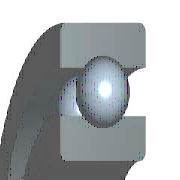
# Autodesk Inventor part: DIN 625 T1 - 619/6 - 6 x 15 x 5
Saved by Autodesk Inventor 2016 (Build 200138000, 138)
## iProperties
IsCustomPart: 0
Created: 2015-02-19
Part Number: DIN 625 T1 - 619/6 - 6 x 15 x 5
Material: Stahl, weich
Description: Rillenkugellager
Document SubType Name: Modeling
Standard: DIN 625 T1
Designer: 4ndreas
Standard Revision: 2011-04
Standards Organization: DIN
Language: de-DE
Size Designation: 619/6 - 6 x 15 x 5
Categories: <MemberInstance><Categories><Category DisplayName="Wellenteile" InternalName="7f7aeb1f-a693-4053-b835-cee3144e0d98" Mnemonic="SHFT"><Category DisplayName="Lager" InternalName="242d30a3-7172-44e6-a363-b0a3d8f1b556" Mnemonic="BRNG"><CategoryParameter DisplayName="Breite" InternalName="25fc5f6e-338b-4801-b5ed-8959743e396e" Mnemonic="wdth"/><CategoryParameter DisplayName="Größenbezeichnung" InternalName="2c4e891a-c8f4-49ed-a5c1-5131476c6feb" Mnemonic="sizedes"/><CategoryParameter DisplayName="Allgemeine Bewertung für dyn. Belastung" InternalName="440972dd-7009-4861-bd45-69ffbb461423" Mnemonic="bdynlrat"/><CategoryParameter DisplayName="Wellendurchmesser" InternalName="91302473-2833-4451-a660-c5d4a8d6a031" Mnemonic="shaftdia"/><CategoryParameter DisplayName="Berührungswinkel" InternalName="aa21a452-7974-4a55-b5cf-1c2972de2aea" Mnemonic="TouchAngle"/><CategoryParameter DisplayName="Außendurchmesser" InternalName="d441686c-04bd-4681-b674-94fbc173ec23" Mnemonic="outdia"/><Category DisplayName="Kugellager" InternalName="9b553946-0899-4a5e-a403-c1d9295e77c1" Mnemonic="BALLBEAR"><CategoryParameter DisplayName="Koeffizient für dynamische Radialbelastung bei Fa/Fr &lt;= e" InternalName="051e59b3-bd55-4dad-8b07-38b5cb912881" Mnemonic="raddynfc1"/><CategoryParameter DisplayName="Allgemeine Bewertung für statische Belastung" InternalName="0f13fbbf-c511-4d43-b4c7-197b47424baf" Mnemonic="bstatlrat"/><CategoryParameter DisplayName="Exponent zur Haltbarkeitsbestimmung" InternalName="3029e2ef-9460-4be8-bdfd-dfe61437473d" Mnemonic="lifeexp"/><CategoryParameter DisplayName="Reibungsfaktor" InternalName="3086b0f2-3d69-46ff-8a75-fe12e395bb47" Mnemonic="fricfct"/><CategoryParameter DisplayName="Min. Wellendurchmesser" InternalName="4a5be9bc-ad86-4bf2-8167-102dad5d3e27" Mnemonic="minshaftdia"/><CategoryParameter DisplayName="Koeffizient für dynamische Axialbelastung bei Fa/Fr &gt; e" InternalName="4b6ff741-5956-4a40-80f5-34eb9259f88c" Mnemonic="axdynfc2"/><CategoryParameter DisplayName="Höchstgeschwindigkeit für Schmierfett" InternalName="5237843b-2c8d-46d3-8227-f3e9dd85a12e" Mnemonic="lubgrsp"/><CategoryParameter DisplayName="Höchstgeschwindigkeit für Öl" InternalName="60628548-8907-44dc-8e09-603d72f5766f" Mnemonic="oilspd"/><CategoryParameter DisplayName="Koeffizient für statische Axialbelastung" InternalName="74dbf5e2-8362-409a-802f-3c2235668d99" Mnemonic="axdynfc0"/><CategoryParameter DisplayName="Masse" InternalName="7b80f85c-da81-4dea-b8db-d7c689da91b2" Mnemonic="mass"/><CategoryParameter DisplayName="Radius" InternalName="83352640-dfae-4cba-bc9f-11ecbfb0001c" Mnemonic="rad"/><CategoryParameter DisplayName="Koeffizient für statische Radialbelastung" InternalName="83ce084d-c51e-4598-a871-e8e1e34b26ee" Mnemonic="raddynfc0"/><CategoryParameter DisplayName="Koeffizient für dynamische Axialbelastung bei Fa/Fr &lt;= e" InternalName="ae45a7db-08df-4411-99a8-2f035015bff9" Mnemonic="axdynfc1"/><CategoryParameter DisplayName="Max. Nabendurchmesser" InternalName="b5cf89e0-ca87-439c-b08c-a25e2999ab06" Mnemonic="maxhubdia"/><CategoryParameter DisplayName="Höchstwert für Faktorbestimmung" InternalName="be0ce6fc-cad4-4218-b484-c34dd2571812" Mnemonic="limvalfac"/><CategoryParameter DisplayName="Koeffizient für dynamische Radialbelastung bei Fa/Fr &gt; e" InternalName="e513bdb7-139f-4b3c-af32-49e0ba1226b9" Mnemonic="raddynfc2"/><CategoryParameter DisplayName="Max. Rundungsradius" InternalName="f6ce6695-cf2c-4ec9-8d20-66671e0e35a4" Mnemonic="maxstprad"/><Category DisplayName="Rillenkugellager" InternalName="6f040212-0f73-4fa8-b5e4-17d6525fdc38" Mnemonic="BBDGBB"/></Category></Category></Category><Category DisplayName="Datentyp" InternalName="23b78d0f-2648-40c6-8793-ca6db495c9e8" Mnemonic="DATATYPE"><CategoryParameter DisplayName="Anzeigename" InternalName="05415f3d-3907-474b-a020-eb9d644f4cf3" Mnemonic="DISPLAYNAME"/><CategoryParameter DisplayName="Norm" InternalName="0c0a119c-1e12-4c84-803f-101930972f5e" Mnemonic="STANDARD"/><CategoryParameter DisplayName="Beschreibung" InternalName="13903e3d-64b1-4950-80da-f627842ea37f" Mnemonic="DESCRIPTION"/><CategoryParameter DisplayName="Bezeichnung" InternalName="2675968c-4ce5-49e0-a4f5-552d29089031" Mnemonic="DESIGNATION"/><CategoryParameter DisplayName="Standardzeile" InternalName="2af9ec52-faaa-4026-b378-f9fa4afca842" Mnemonic="DEFAULTROW"/><CategoryParameter DisplayName="Ordnername" InternalName="3f06958e-8713-4116-9be7-ed6184ecc97b" Mnemonic="FOLDERNAME"/><CategoryParameter DisplayName="Revisionsanleitung" InternalName="45a75005-10b1-4dfc-8d6d-dfe629f0b93c" Mnemonic="REVISIONGUID"/><CategoryParameter DisplayName="Dateiname" InternalName="8b46a4cc-9585-4fed-90c3-899f57e09a73" Mnemonic="FILENAME"/><CategoryParameter DisplayName="Normungsorganisation" InternalName="8f5914e1-4693-403f-8ab5-d37768198c9d" Mnemonic="STDSORG"/><CategoryParameter DisplayName="Gruppenversion" InternalName="914462f6-6e19-4b14-ba84-155b9680b1d0" Mnemonic="FAMILYREVISION"/><CategoryParameter DisplayName="Normrevision" InternalName="91d5a463-65c2-4fde-b823-3b7fea5e8e17" Mnemonic="STANDARDREVISION"/><CategoryParameter DisplayName="Variantenrevision" InternalName="a65d44b9-392f-4f4f-857b-e4b3d54996fe" Mnemonic="MEMBERREVISION"/><CategoryParameter DisplayName="ClipFormat" InternalName="bc51e27b-3422-4e78-93ef-cec197ddf230" Mnemonic="CLIPFORMAT"/><CategoryParameter DisplayName="Hersteller" InternalName="cd6c7a72-a28a-4e50-99a9-2c7f4e13e5ad" Mnemonic="MANUFACTURER"/><CategoryParameter DisplayName="InternerName" InternalName="cf1d0246-76d9-4b4a-8305-fa0409afb5c1" Mnemonic="INTERNALNAME"/><CategoryParameter DisplayName="IstMetrisch" InternalName="e2385c5b-1ea4-4823-96a8-8de651266ec3" Mnemonic="ISMETRIC"/><Category DisplayName="Bauteil" InternalName="c0e0b642-3bcb-4cc8-9e80-f96d35c4afa4" Mnemonic="PART"><CategoryParameter DisplayName="Bauteilnummer" InternalName="016b6077-bfbe-49bd-92c9-d8d59c39c941" Mnemonic="PARTNUMBER"/><CategoryParameter DisplayName="Bestandsnummer" InternalName="4dba7c1c-e26c-444e-836c-b08b433409a8" Mnemonic="STOCKNUMBER"/><CategoryParameter DisplayName="Materialschlüssel" InternalName="5c9a8adb-dd2b-4535-b97f-0a94a95fe41f" Mnemonic="MATERIALKEY"/><CategoryParameter DisplayName="Material" InternalName="818a152a-d3c3-49ca-80ee-df7d91421b8e" Mnemonic="MATERIAL"/></Category></Category><Category DisplayName="ÄltereVersionenzuweisen" InternalName="cd87c42b-3e48-431e-b5c0-1cbeb14dfe77" Mnemonic="LEGACYMAP"><CategoryParameter DisplayName="Eindeutige DA-Varianten-ID" InternalName="0918ad47-427f-4fed-ae26-24c81c58f590" Mnemonic="DACOOKIE"/><CategoryParameter DisplayName="ID zusammenführen" InternalName="0ee8fb18-e2ed-4f39-96f6-1f4b5f50aa71" Mnemonic="MERGE11"/><CategoryParameter DisplayName="Eindeutige CC-Varianten-ID" InternalName="5193edd4-b2b0-4ab4-9d54-de900eee34e0" Mnemonic="CCCOOKIE"/><CategoryParameter DisplayName="ID aufteilen" InternalName="72b5c83c-be7f-45c4-ae51-9160ea6deb26" Mnemonic="SPLIT"/><CategoryParameter DisplayName="VarianteID" InternalName="8e5e0294-fc51-4c8f-b3d7-003dc5ed94f6" Mnemonic="MEMBERID"/><CategoryParameter DisplayName="Katalogname" InternalName="d99d1e27-aa94-4de2-af4c-c348882a6f4f" Mnemonic="CATALOGNAME"/><CategoryParameter DisplayName="Gruppennummer" InternalName="e705e1f4-09cb-413e-91f9-551b4188271e" Mnemonic="FAMILYNUMBER"/></Category></Categories><FamilyTemplate Id="br0026"><FamilyTemplateParameters><FamilyTemplateParameter ObjectType="kUserParameterObject" ValueType="xs:double" Id="1" ObjectReferenceKey="WR"/><FamilyTemplateParameter ObjectType="kUserParameterObject" ValueType="xs:double" Id="2" ObjectReferenceKey="DDB"/><FamilyTemplateParameter ObjectType="kUserParameterObject" ValueType="xs:double" Id="3" ObjectReferenceKey="DDA"/><FamilyTemplateParameter ObjectType="kUserParameterObject" ValueType="xs:double" Id="4" ObjectReferenceKey="KRS"/><FamilyTemplateParameter ObjectType="kUserParameterObject" ValueType="xs:double" Id="5" ObjectReferenceKey="WD"/><FamilyTemplateParameter ObjectType="kUserParameterObject" ValueType="xs:double" Id="6" ObjectReferenceKey="KAD1"/><FamilyTemplateParameter ObjectType="kUserParameterObject" ValueType="xs:double" Id="7" ObjectReferenceKey="KB"/><FamilyTemplateParameter ObjectType="kUserParameterObject" ValueType="xs:double" Id="8" ObjectReferenceKey="BC0"/><FamilyTemplateParameter ObjectType="kUserParameterObject" ValueType="xs:double" Id="9" ObjectReferenceKey="BD"/><FamilyTemplateParameter ObjectType="kUserParameterObject" ValueType="xs:double" Id="10" ObjectReferenceKey="BC"/><FamilyTemplateParameter ObjectType="kUserParameterObject" ValueType="xs:double" Id="11" ObjectReferenceKey="BR"/><FamilyTemplateParameter ObjectType="kUserParameterObject" ValueType="xs:double" Id="12" ObjectReferenceKey="BBA"/><FamilyTemplateParameter ObjectType="kUserParameterObject" ValueType="xs:double" Id="13" ObjectReferenceKey="KID1"/><FamilyTemplateParameter ObjectType="kUserParameterObject" ValueType="xs:double" Id="14" ObjectReferenceKey="BI"/><FamilyTemplateParameter ObjectType="kPropertyObject" ValueType="xs:string" Id="100" ObjectReferenceKey="{32853F0F-3444-11d1-9E93-0060B03C1CA6}" SubObjectId="52"/><FamilyTemplateParameter ObjectType="kPropertyObject" ValueType="xs:string" Id="105" ObjectReferenceKey="{32853F0F-3444-11d1-9E93-0060B03C1CA6}" SubObjectId="5"/><FamilyTemplateParameter ObjectType="kPartComponentDefinitionObject" ValueType="xs:string" Id="110" SubObjectId="Material"/></FamilyTemplateParameters></FamilyTemplate><CategoryParameterMap><ParamToTemplateMap><ParamToTemplate CategoryParameter="//CategoryParameter[@InternalName='05415f3d-3907-474b-a020-eb9d644f4cf3']" ConstantValue="DIN 625 - T1"/><ParamToTemplate CategoryParameter="//CategoryParameter[@InternalName='cf1d0246-76d9-4b4a-8305-fa0409afb5c1']" ConstantValue="5d4a6c16-d65c-4e33-9660-dc348c1d9e25"/><ParamToTemplate CategoryParameter="//CategoryParameter[@InternalName='3f06958e-8713-4116-9be7-ed6184ecc97b']" ConstantValue="DIN 625 - T1"/><ParamToTemplate CategoryParameter="//CategoryParameter[@InternalName='914462f6-6e19-4b14-ba84-155b9680b1d0']" ConstantValue="10"/><ParamToTemplate CategoryParameter="//CategoryParameter[@InternalName='bc51e27b-3422-4e78-93ef-cec197ddf230']" ConstantValue="CF_INVENTOR.STDPARTS"/><ParamToTemplate CategoryParameter="//CategoryParameter[@InternalName='e2385c5b-1ea4-4823-96a8-8de651266ec3']" ConstantValue="true"/><ParamToTemplate CategoryParameter="//CategoryParameter[@InternalName='13903e3d-64b1-4950-80da-f627842ea37f']" ConstantValue="Deep Groove Ball Bearing"/><ParamToTemplate CategoryParameter="//CategoryParameter[@InternalName='8f5914e1-4693-403f-8ab5-d37768198c9d']" ConstantValue="DIN"/><ParamToTemplate CategoryParameter="//CategoryParameter[@InternalName='0c0a119c-1e12-4c84-803f-101930972f5e']" ConstantValue="DIN 625 T1"/><ParamToTemplate CategoryParameter="//CategoryParameter[@InternalName='cd6c7a72-a28a-4e50-99a9-2c7f4e13e5ad']" TemplateParameter="104"/><ParamToTemplate CategoryParameter="//CategoryParameter[@InternalName='91d5a463-65c2-4fde-b823-3b7fea5e8e17']" ConstantValue="2011-04"/><ParamToTemplate CategoryParameter="//CategoryParameter[@InternalName='45a75005-10b1-4dfc-8d6d-dfe629f0b93c']" ConstantValue="d6feace9-0a94-4a7e-876f-687225c7e903"/><ParamToTemplate CategoryParameter="//CategoryParameter[@InternalName='2af9ec52-faaa-4026-b378-f9fa4afca842']" ConstantValue="10"/><ParamToTemplate CategoryParameter="//CategoryParameter[@InternalName='d99d1e27-aa94-4de2-af4c-c348882a6f4f']" ConstantValue="DIN"/><ParamToTemplate CategoryParameter="//CategoryParameter[@InternalName='e705e1f4-09cb-413e-91f9-551b4188271e']" ConstantValue="249"/><ParamToTemplate CategoryParameter="//CategoryParameter[@InternalName='8b46a4cc-9585-4fed-90c3-899f57e09a73']" ConstantValue="DIN 625 T1 - 619/6 - 6 x 15 x 5"/><ParamToTemplate CategoryParameter="//CategoryParameter[@InternalName='a65d44b9-392f-4f4f-857b-e4b3d54996fe']" ConstantValue="51BD74BC-A623-4305-A976-BDE71F3737EF"/><ParamToTemplate CategoryParameter="//CategoryParameter[@InternalName='2c4e891a-c8f4-49ed-a5c1-5131476c6feb']" ConstantValue="619/6"/><ParamToTemplate CategoryParameter="//CategoryParameter[@InternalName='8e5e0294-fc51-4c8f-b3d7-003dc5ed94f6']" ConstantValue="2400"/><ParamToTemplate CategoryParameter="//CategoryParameter[@InternalName='aa21a452-7974-4a55-b5cf-1c2972de2aea']" TemplateParameter="12"/><ParamToTemplate CategoryParameter="//CategoryParameter[@InternalName='440972dd-7009-4861-bd45-69ffbb461423']" TemplateParameter="10"/><ParamToTemplate CategoryParameter="//CategoryParameter[@InternalName='0f13fbbf-c511-4d43-b4c7-197b47424baf']" TemplateParameter="8"/><ParamToTemplate CategoryParameter="//CategoryParameter[@InternalName='d441686c-04bd-4681-b674-94fbc173ec23']" TemplateParameter="9"/><ParamToTemplate CategoryParameter="//CategoryParameter[@InternalName='2675968c-4ce5-49e0-a4f5-552d29089031']" TemplateParameter="100"/><ParamToTemplate CategoryParameter="//CategoryParameter[@InternalName='25fc5f6e-338b-4801-b5ed-8959743e396e']" TemplateParameter="7"/><ParamToTemplate CategoryParameter="//CategoryParameter[@InternalName='83352640-dfae-4cba-bc9f-11ecbfb0001c']" TemplateParameter="4"/><ParamToTemplate CategoryParameter="//CategoryParameter[@InternalName='818a152a-d3c3-49ca-80ee-df7d91421b8e']" TemplateParameter="110"/><ParamToTemplate CategoryParameter="//CategoryParameter[@InternalName='016b6077-bfbe-49bd-92c9-d8d59c39c941']" TemplateParameter="105"/><ParamToTemplate CategoryParameter="//CategoryParameter[@InternalName='91302473-2833-4451-a660-c5d4a8d6a031']" TemplateParameter="5"/></ParamToTemplateMap></CategoryParameterMap></MemberInstance>
Density: 7.85 g/cm^3
Appearance: Halbpoliert
Mass: 1.68915 g
Surface Area: 6.84168 cm^2
Volume: 0.215178 cm^3
Author: 4ndreas
Autodesk Inventor part; units mm, degrees
note: some values were not read from the file. Left out: dimensions or parameters whose unit could not be read.
ref_plane "YZ Plane" through (0, 0, 0) normal (1, 0, 0) x (0, 1, 0)
ref_plane "XZ Plane" through (0, 0, 0) normal (0, 1, 0) x (-1, 0, 0)
ref_plane "XY Plane" through (0, 0, 0) normal (0, 0, 1) x (1, 0, 0)
sketch "Skizze" plane through (0, 0, 0) normal (0, 0, 1) x (1, 0, 0)
  circle A0 centre (2.5, 4.25) radius 0.75
  line L0 (1.75, 4.25) -> (3.25, 4.25)
  line L1 (2.5, 4.25) -> (2.5, 3.5)
  line L2 (1.9, 3.8) -> (0, 3.8)
  line L3 (0, 3) -> (5, 3)
  line L4 (1.9, 4.7) -> (0, 4.7)
  line L5 (0, 5.5) -> (5, 5.5)
  line L6 (3.1, 3.8) -> (5, 3.8)
  line L7 (3.1, 4.7) -> (5, 4.7)
  line L8 (5, 4.7) -> (5, 5.5)
  line L9 (5, 3) -> (5, 3.8)
  line L10 (2.5, 4.25) -> (2.5, 5)
  line L11 (-1, 0) -> (6, 0) projected
  line L12 (0, 2.1) -> (0, 8.4) projected
  dimension "d3" = 1.5
  dimension "d8" = 6
  dimension "d10" = 7.6
  dimension "d12" = 9.4
  dimension "d13" = 11
  dimension "d14" = 8.5
  dimension "d15" = 5
  constraints: 22 end point, 4 point on line, 3 parallel, 3 perpendicular, 3 symmetric about line, 1 midpoint, 12 other
  measures "d8" diameter of L3 L11
  measures "d10" diameter of L2 L11
  measures "d12" diameter of L4 L11
  measures "d13" diameter of L5 L11
  measures "d14" diameter of L1.start L11
  measures "d15" distance between parallel lines of L12 L9
revolve "Körper" add sketch "Skizze" angle 360 about axis through (-10, 0, 0) along (1, 0, 0) contours A0 L4 L12 L5 L8 L7 | L6 L9 L3 L12 L2 A0
fillet "Rundung1" radius 0.2 4 edges at (5, -3, 0) (0, -3, 0) (0, -5.5, 0) (5, -5.5, 0)
revolve "Kugel" add sketch "Skizze" angle 360 about axis through (1.75, 4.25, 0) along (1, 0, 0) contours A0 L1 L0 | L1 A0 L0
pattern_circular "Kugeln" count 9 over 360 about axis through (-10, 0, 0) along (1, 0, 0) of "Kugel"
equation "\"d3\" = DDB"
equation "\"d8\" = WD"
equation "\"d10\" = KID1"
equation "\"d12\" = KAD1"
equation "\"d13\" = BD"
equation "\"d14\" = DDA"
equation "\"d15\" = KB"
equation "\"d0\" = KRS"
equation "\"WD\" = 6"
equation "\"BD\" = 11"
equation "\"KB\" = 5"
equation "\"KRS\" = 0.2"
equation "\"KID1\" = DDA - 0.6 * DDB"
equation "\"KAD1\" = DDA + 0.6 * DDB"
equation "\"DDA\" = 0.5 * WD + 0.5 * BD"
equation "\"DDB\" = -0.3 * WD + 0.3 * BD"
equation "\"WR\" = 0.5 * WD"
equation "\"BR\" = 0.5 * BD"
equation "\"BBA\" = 0"
body "Solid1"
